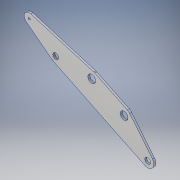
# Autodesk Inventor part: Intake Arm
Saved by Autodesk Inventor 2019.4 (Build 234330000, 330)
## iProperties
Created: 2020-01-27
Part Number: Intake Arm
Material: Aluminum 6061
Document SubType Name: Modeling
Designer: admin
Density: 2.7 g/cm^3
Appearance: Aluminum - Flat
Author: admin
Autodesk Inventor part; units mm, degrees
ref_plane "YZ Plane" through (0, 0, 0) normal (1, 0, 0) x (0, 1, 0)
ref_plane "XZ Plane" through (0, 0, 0) normal (0, 1, 0) x (-1, 0, 0)
ref_plane "XY Plane" through (0, 0, 0) normal (0, 0, 1) x (1, 0, 0)
sketch "Sketch1" plane through (0, 0, 0) normal (0, 0, 1) x (1, 0, 0)
  circle A0 centre (0, 0) radius 7
  circle A1 centre (224.8886, -109.2022) radius 7
  line L0 (224.8886, -109.2022) -> (0, 0) construction
  line L1 (-22.292, -122) -> (120, -122) construction
  line L2 (120, -122) -> (120, -250) construction
  line L3 (120, -250) -> (-22.292, -250) construction
  line L4 (-22.292, -250) -> (-22.292, -122) construction
  line L5 (-328.9804, -295.7312) -> (1127.5246, -295.7312) construction
  line L6 (-64.1335, -215.7312) -> (38.7642, -215.7312)
  line L7 (38.7642, -215.7312) -> (38.7642, -252.1222)
  circle A2 centre (224.8886, -109.2022) radius 50 construction
  circle A3 centre (88.0787, -3.8614) radius 9.5
  circle A4 centre (88.0787, -3.8614) radius 25.4 construction
  circle A5 centre (167.3865, -42.3719) radius 9.5
  circle A6 centre (167.3865, -42.3719) radius 25.4 construction
  line L8 (88.0787, -3.8614) -> (0, 0) construction
  line L9 (88.0787, -3.8614) -> (167.3865, -42.3719) construction
  line L10 (167.3865, -42.3719) -> (224.8886, -109.2022) construction
  circle A7 centre (-64.803, 46.9103) radius 2.5
  line L11 (-64.803, 46.9103) -> (0, 0) construction
  circle A8 centre (146.9957, -220.6144) radius 88.9 construction
  arc A9 (-6.5521, -13.4933) -> (-9.1711, -11.8697) centre (0, 0) ccw construction
  arc A10 (236.5319, -99.7452) -> (218.3365, -122.6955) centre (224.8886, -109.2022) ccw construction
  line L12 (-72.3831, 36.9708) -> (-9.1711, -11.8697)
  arc A11 (-9.1711, -11.8697) -> (-6.5521, -13.4933) centre (0, 0) ccw
  arc A12 (218.3365, -122.6955) -> (236.5319, -99.7452) centre (224.8886, -109.2022) ccw
  arc A13 (93.0761, 12.9099) -> (95.7229, 11.8808) centre (88.0787, -3.8614) ccw construction
  arc A14 (95.7229, 11.8808) -> (93.0761, 12.9099) centre (88.0787, -3.8614) ccw
  line L13 (-6.5521, -13.4933) -> (218.3365, -122.6955)
  arc A15 (175.0306, -26.6297) -> (180.9703, -31.3388) centre (167.3865, -42.3719) ccw construction
  line L14 (180.9703, -31.3388) -> (236.5319, -99.7452)
  line L15 (175.0306, -26.6297) -> (95.7229, 11.8808)
  arc A16 (180.9703, -31.3388) -> (175.0306, -26.6297) centre (167.3865, -42.3719) ccw
  arc A17 (-72.3831, 36.9708) -> (-61.2334, 58.8898) centre (-64.803, 46.9103) ccw construction
  line L16 (-61.2334, 58.8898) -> (93.0761, 12.9099)
  arc A18 (-61.2334, 58.8898) -> (-72.3831, 36.9708) centre (-64.803, 46.9103) ccw
  dimension "d0" = 14
  dimension "d3" = 14
  dimension "d4" = 250
  dimension "d5" = 120
  dimension "d6" = 128
  dimension "d7" = 122
  dimension "d9" = 80
  dimension "d11" = 100
  dimension "d12" = 19
  dimension "d15" = 19
  dimension "d16" = 50.8
  dimension "d17" = 50.8
  dimension "d18" = 35
  dimension "d19" = 35
  dimension "d20" = 5
  dimension "d22" = 80
  dimension "d23" = 170
  dimension "d24" = 177.8
  dimension "d28" = 30
  dimension "d31" = 30
  dimension "d32" = 35
  dimension "d33" = 35
  dimension "d34" = 25
  constraints: 34 end point, 20 point on circle, 19 centre point, 11 coincident, 9 tangent, 3 horizontal, 3 perpendicular, 2 equal length, 2 parallel
  measures "d0" diameter of A0
  measures "d3" diameter of A1
  measures "d4" distance of L0.start L0.end
  measures "d5" distance from line of L0.end L2
  measures "d6" distance of L3.end L1.start
  measures "d7" distance from line of A0.centre L1
  measures "d9" distance between parallel lines of L5 L6
  measures "d11" diameter of A2
  measures "d12" diameter of A3
  measures "d15" diameter of A5
  measures "d16" diameter of A6
  measures "d17" diameter of A4
  measures "d18" distance from line of L0 A3.centre
  measures "d19" distance from line of L0 L9.end
  measures "d20" diameter of A7
  measures "d22" distance of L11.start L0.end
  measures "d23" angle of L0 L11
  measures "d24" diameter of A8
  measures "d28" diameter of A9
  measures "d31" diameter of A10
  measures "d32" diameter of A13
  measures "d33" diameter of A15
  measures "d34" diameter of A17
extrude "Extrusion1" add sketch "Sketch1" along normal blind 5
body "Solid1"
